Autodesk Fusion 360 part; units mm, degrees
note: some values were not read from the file. Set by a fixed rule: which face or edge a step refers to.
(part 5 of 5)
sketch "Sketch1" plane through (0, 0, 0) normal (0, 0, 1) x (1, 0, 0)
  line L0 (-10, 10) -> (10, 10) construction
  line L1 (10, 10) -> (10, -10) construction
  line L2 (10, -10) -> (-10, -10) construction
  line L3 (-10, -10) -> (-10, 10) construction
  circle A0 centre (0, 0) radius 2.5
  line L4 (0, -10) -> (0, -3.9) construction
  line L5 (-10, 0) -> (-3.9, 0) construction
  line L6 (10, 0) -> (3.9, 0) construction
  line L7 (0, 10) -> (0, 3.9) construction
  line L8 (3.9, 3.6) -> (3.9, 0) construction
  line L9 (3.9, -3.0515) -> (3.9, 3.1)
  line L10 (-3.9, 3.1) -> (-3.9, -3.0515)
  line L11 (10, 10) -> (-10, -10) construction
  line L12 (-10, 10) -> (10, -10) construction
  line L13 (3.9, 3.9) -> (4.3243, 3.4757) construction
  line L14 (3.9, 3.9) -> (3.4757, 4.3243) construction
  line L15 (-3.9, 3.9) -> (-3.4757, 4.3243) construction
  line L16 (-3.4757, 4.3243) -> (-4.3243, 3.4757) construction
  line L17 (-3.9, -3.9) -> (-4.3243, -3.4757) construction
  line L18 (-4.3243, -3.4757) -> (-3.4757, -4.3243) construction
  line L19 (3.9, -3.9) -> (4.3243, -3.4757) construction
  line L20 (4.3243, -3.4757) -> (3.4757, -4.3243) construction
  line L21 (3.4757, -4.3243) -> (3.0515, -3.9)
  line L22 (4.3243, -3.4757) -> (3.9, -3.0515)
  line L23 (10, -10) -> (9.1515, -10)
  line L24 (10, -9.1515) -> (10, -10)
  line L25 (3.4757, 4.3243) -> (3.0515, 3.9)
  line L26 (3.4757, 4.3243) -> (2.8757, 4.3243) construction
  line L27 (4.3243, 3.4757) -> (3.9, 3.0515)
  line L28 (-4.3243, 3.4757) -> (-3.9, 3.0515)
  line L29 (-3.4757, 4.3243) -> (-3.0515, 3.9)
  line L30 (-3.4757, -4.3243) -> (-3.0515, -3.9)
  line L31 (-4.3243, -3.4757) -> (-3.9, -3.0515)
  line L32 (-4.3243, -3.4757) -> (-3.7243, -3.4757) construction
  line L33 (-9.1515, -10) -> (-10, -10)
  line L34 (-10, -10) -> (-10, -9.1515)
  line L35 (-10, 9.1515) -> (-10, 10)
  line L36 (-10, 10) -> (-9.1515, 10)
  line L37 (9.1515, 10) -> (10, 10)
  line L38 (10, 9.1515) -> (10, 10)
  line L39 (10, -10) -> (8.2, -10) construction
  line L40 (8.2, -10) -> (8.2, -8.2) construction
  line L41 (8.2, -8.2) -> (10, -8.2) construction
  line L42 (10, -8.2) -> (10, -10) construction
  line L43 (-10, -10) -> (-8.2, -10) construction
  line L44 (-8.2, -10) -> (-8.2, -8.2) construction
  line L45 (-8.2, -8.2) -> (-10, -8.2) construction
  line L46 (-10, -8.2) -> (-10, -10) construction
  line L47 (-10, 10) -> (-8.2, 10) construction
  line L48 (-8.2, 10) -> (-8.2, 8.2) construction
  line L49 (-8.2, 8.2) -> (-10, 8.2) construction
  line L50 (-10, 8.2) -> (-10, 10) construction
  line L51 (10, 10) -> (8.2, 10) construction
  line L52 (8.2, 10) -> (8.2, 8.2) construction
  line L53 (8.2, 8.2) -> (10, 8.2) construction
  line L54 (10, 8.2) -> (10, 10) construction
  line L55 (-10, -10) -> (-9.1, -10) construction
  line L56 (-9.1, -10) -> (-9.1, -9.1) construction
  line L57 (-9.1, -9.1) -> (-10, -9.1) construction
  line L58 (-10, -9.1) -> (-10, -10) construction
  line L59 (-10, 10) -> (-9.1, 10) construction
  line L60 (-9.1, 10) -> (-9.1, 9.1) construction
  line L61 (-9.1, 9.1) -> (-10, 9.1) construction
  line L62 (-10, 9.1) -> (-10, 10) construction
  line L63 (10, 10) -> (9.1, 10) construction
  line L64 (9.1, 10) -> (9.1, 9.1) construction
  line L65 (9.1, 9.1) -> (10, 9.1) construction
  line L66 (10, 9.1) -> (10, 10) construction
  line L67 (10, -10) -> (9.1, -10) construction
  line L68 (9.1, -10) -> (9.1, -9.1) construction
  line L69 (9.1, -9.1) -> (10, -9.1) construction
  line L70 (10, -9.1) -> (10, -10) construction
  line L71 (0, -10) -> (3.1, -10) construction
  line L72 (3.1, -10) -> (-3, -10) construction
  line L73 (-3, -10) -> (-3, 10) construction
  line L74 (-3, 10) -> (3.1, 10) construction
  line L75 (3.1, 10) -> (3.1, -10) construction
  line L76 (-10, 0) -> (-10, 3.1) construction
  line L77 (-10, 3.1) -> (10, 3.1) construction
  line L78 (10, 3.1) -> (10, -3) construction
  line L79 (10, -3) -> (-10, -3) construction
  line L80 (-10, -3) -> (-10, 3.1) construction
  line L81 (0, -10) -> (-5.45, -10) construction
  line L82 (-5.45, -10) -> (5.45, -10) construction
  line L83 (5.45, 10) -> (-5.45, 10) construction
  line L84 (-10, 0) -> (-10, 5.45) construction
  line L85 (10, 5.45) -> (10, -5.45) construction
  line L86 (-10, -5.45) -> (-10, 5.45) construction
  line L87 (-10, -10) -> (-5.45, -10)
  line L88 (-10, -5.45) -> (-10, -10)
  line L89 (10, -10) -> (5.45, -10)
  line L90 (10, -5.45) -> (10, -10)
  line L91 (10, 10) -> (5.45, 10)
  line L92 (5.45, 8.2) -> (5.45, 6.2985)
  line L93 (10, 5.45) -> (10, 10)
  line L94 (-10, 10) -> (-5.45, 10)
  line L95 (-5.45, 8.2) -> (-5.45, 6.2985)
  line L96 (-6.2985, 5.45) -> (-8.2, 5.45)
  line L97 (-10, 5.45) -> (-10, 10)
  line L98 (10, 0) -> (10, 3.6) construction
  line L99 (-10, 3.6) -> (-10, -3.6) construction
  line L100 (10, -3.6) -> (10, 3.6) construction
  line L101 (0, 10) -> (-3.6, 10) construction
  line L102 (-3.6, 10) -> (3.6, 10) construction
  line L103 (3.6, -10) -> (-3.6, -10) construction
  line L104 (-8.2, -8.2) -> (8.2, -8.2) construction
  line L105 (8.2, -8.2) -> (8.2, 8.2) construction
  line L106 (8.2, 8.2) -> (-8.2, 8.2) construction
  line L107 (-8.2, 8.2) -> (-8.2, -8.2) construction
  line L108 (-5.45, -10) -> (-3.6, -10)
  line L109 (-3.6, -10) -> (-3.6, -9.1)
  line L110 (-3.6, -8.2) -> (-5.45, -8.2)
  line L111 (-10, -3.6) -> (-9.1, -3.6)
  line L112 (-8.2, -3.6) -> (-8.2, -5.45)
  line L113 (-10, -5.45) -> (-10, -3.6)
  line L114 (-9.1, 3.6) -> (-10, 3.6)
  line L115 (-10, 3.6) -> (-10, 5.45)
  line L116 (-8.2, 5.45) -> (-8.2, 3.6)
  line L117 (3.6, 8.2) -> (5.45, 8.2)
  line L118 (5.45, 10) -> (3.6, 10)
  line L119 (3.6, 10) -> (3.6, 9.1)
  line L120 (-5.45, 10) -> (-3.6, 10)
  line L121 (-3.6, 10) -> (-3.6, 9.1)
  line L122 (-3.6, 8.2) -> (-5.45, 8.2)
  line L123 (10, 5.45) -> (10, 3.6)
  line L124 (10, 3.6) -> (9.1, 3.6)
  line L125 (8.2, 3.6) -> (8.2, 5.45)
  line L126 (10, -5.45) -> (10, -3.6)
  line L127 (10, -3.6) -> (9.1, -3.6)
  line L128 (8.2, -3.6) -> (8.2, -5.45)
  line L129 (5.45, -8.2) -> (3.6, -8.2)
  line L130 (3.6, -9.1) -> (3.6, -10)
  line L131 (3.6, -10) -> (5.45, -10)
  line L132 (9.1, -9.1) -> (-9.1, -9.1) construction
  line L133 (-9.1, -9.1) -> (-9.1, 9.1) construction
  line L134 (-9.1, 9.1) -> (9.1, 9.1) construction
  line L135 (9.1, 9.1) -> (9.1, -9.1) construction
  line L136 (3.6, -9.1) -> (3.1, -9.1)
  line L137 (3.1, -9.1) -> (3.1, -8.2)
  line L138 (3.1, -8.2) -> (3.6, -8.2)
  line L139 (-3, -9.1) -> (-3.6, -9.1)
  line L140 (-3.6, -8.2) -> (-3, -8.2)
  line L141 (-3, -8.2) -> (-3, -9.1)
  line L142 (-8.2, -3.6) -> (-8.2, -3)
  line L143 (-8.2, -3) -> (-9.1, -3)
  line L144 (-9.1, -3) -> (-9.1, -3.6)
  line L145 (-8.2, 3.6) -> (-8.2, 3.1)
  line L146 (-8.2, 3.1) -> (-9.1, 3.1)
  line L147 (-9.1, 3.1) -> (-9.1, 3.6)
  line L148 (-3.6, 9.1) -> (-3, 9.1)
  line L149 (-3, 9.1) -> (-3, 8.2)
  line L150 (-3, 8.2) -> (-3.6, 8.2)
  line L151 (3.1, 9.1) -> (3.6, 9.1)
  line L152 (3.6, 8.2) -> (3.1, 8.2)
  line L153 (3.1, 8.2) -> (3.1, 9.1)
  line L154 (9.1, 3.6) -> (9.1, 3.1)
  line L155 (9.1, 3.1) -> (8.2, 3.1)
  line L156 (8.2, 3.1) -> (8.2, 3.6)
  line L157 (9.1, -3.6) -> (9.1, -3)
  line L158 (9.1, -3) -> (8.2, -3)
  line L159 (8.2, -3) -> (8.2, -3.6)
  line L160 (-3.4757, 4.3243) -> (-5.45, 6.2985)
  line L161 (-4.3243, 3.4757) -> (-6.2985, 5.45)
  line L162 (-3.6, 9.1) -> (-3.6, 10) construction
  line L163 (-9.1, 3.6) -> (-10, 3.6) construction
  line L164 (-3.0515, -3.9) -> (3.1, -3.9)
  line L165 (-3.9, 0) -> (-3.9, -3.0515) construction
  line L166 (0, 3.9) -> (3.1, 3.9) construction
  line L167 (3.1, 3.9) -> (-3.0515, 3.9)
  line L168 (-4.3243, -3.4757) -> (-6.2985, -5.45)
  line L169 (-3.4757, -4.3243) -> (-5.45, -6.2985)
  line L170 (-6.2985, -5.45) -> (-8.2, -5.45)
  line L171 (-10, -3.6) -> (-9.1, -3.6) construction
  line L172 (-5.45, -8.2) -> (-5.45, -6.2985)
  line L173 (-3.6, -10) -> (-3.6, -9.1) construction
  line L174 (-3.6, -8.2) -> (-3.6, 8.2) construction
  line L175 (6.2985, -5.45) -> (8.2, -5.45)
  line L176 (-8.2, -3.6) -> (8.2, -3.6) construction
  line L177 (9.1, -3.6) -> (10, -3.6) construction
  line L178 (3.4757, -4.3243) -> (5.45, -6.2985)
  line L179 (8.2, -9.0485) -> (8.2515, -9.1)
  line L180 (9.1, -9.9485) -> (9.1515, -10)
  line L181 (9.9485, -9.1) -> (10, -9.1515)
  line L182 (4.3243, -3.4757) -> (6.2985, -5.45)
  line L183 (9.0485, -8.2) -> (9.1, -8.2515)
  line L184 (5.45, -8.2) -> (5.45, -6.2985)
  line L185 (6.2985, 5.45) -> (8.2, 5.45)
  line L186 (10, 3.6) -> (9.1, 3.6) construction
  line L187 (8.2, 3.6) -> (-8.2, 3.6) construction
  line L188 (3.4757, 4.3243) -> (5.45, 6.2985)
  line L189 (4.3243, 3.4757) -> (6.2985, 5.45)
  line L190 (3.6, 10) -> (3.6, 9.1) construction
  line L191 (3.6, 8.2) -> (3.6, -10) construction
  dimension "d1" = 20
  dimension "d2" = 20
  dimension "d3" = 5
  dimension "d4" = 6.1
  dimension "d5" = 6.1
  dimension "d6" = 6.1
  dimension "d7" = 6.1
  dimension "d8" = 0.6
  dimension "d9" = 0.6
  dimension "d10" = 0.6
  dimension "d11" = 1.2
  dimension "d12" = 0.6
  dimension "d13" = 1.2
  dimension "d14" = 0.6
  dimension "d15" = 1.2
  dimension "d18" = 45
  dimension "d20" = 45
  dimension "d24" = 1.8
  dimension "d25" = 1.8
  dimension "d26" = 1.8
  dimension "d27" = 1.8
  dimension "d28" = 1.8
  dimension "d29" = 1.8
  dimension "d30" = 1.8
  dimension "d31" = 1.8
  dimension "d32" = 0.9
  dimension "d33" = 0.9
  dimension "d34" = 0.9
  dimension "d35" = 0.9
  dimension "d36" = 0.9
  dimension "d37" = 0.9
  dimension "d38" = 0.9
  dimension "d39" = 0.9
  dimension "d40" = 3.1
  dimension "d41" = 6.1
  dimension "d42" = 3.1
  dimension "d43" = 20
  dimension "d44" = 6.1
  dimension "d47" = 5.45
  dimension "d48" = 10.9
  dimension "d49" = 3.6
  dimension "d50" = 7.2
  dimension "d51" = 20
  dimension "d52" = 3.6
  dimension "d53" = 7.2
  dimension "d54" = 20
  constraint horizontal L0
  constraint vertical L1
  constraint horizontal L2
  constraint vertical L3
  constraint coincident A0.centre origin
  constraint midpoint L2 L4.start
  constraint perpendicular L2 L4
  constraint midpoint L3 L5.start
  constraint perpendicular L3 L5
  constraint perpendicular L5 L165
  constraint midpoint L1 L6.start
  constraint perpendicular L1 L6
  constraint midpoint L0 L7.start
  constraint perpendicular L0 L7
  constraint perpendicular L7 L166
  constraint perpendicular L6 L8
  constraint vertical L9
  constraint vertical L10
  constraint parallel L12 L13
  constraint perpendicular L11 L14
  constraint perpendicular L12 L15
  constraint perpendicular L12 L16
  constraint perpendicular L11 L17
  constraint perpendicular L11 L18
  constraint perpendicular L12 L19
  constraint perpendicular L12 L20
  constraint coincident L2 L23.end
  constraint perpendicular L20 L178
  constraint perpendicular L20 L21
  constraint perpendicular L19 L22
  constraint coincident L1 L24.start
  constraint perpendicular L19 L182
  constraint perpendicular L1 L23
  constraint perpendicular L2 L24
  constraint coincident L1 L38.start
  constraint coincident L0 L37.start
  constraint horizontal L26
  constraint coincident L25.end L166
  constraint coincident L8 L27.end
  constraint coincident L10 L28.end
  constraint perpendicular L16 L28
  constraint perpendicular L16 L29
  constraint perpendicular L18 L30
  constraint horizontal L32
  constraint coincident L3 L34.end
  constraint perpendicular L17 L168
  constraint coincident L2 L33.start
  constraint perpendicular L33 L34
  constraint coincident L3 L35.start
  constraint coincident L0 L36.end
  constraint horizontal L39
  constraint vertical L40
  constraint horizontal L41
  constraint vertical L42
  constraint horizontal L43
  constraint vertical L44
  constraint horizontal L45
  constraint vertical L46
  constraint horizontal L47
  constraint vertical L48
  constraint horizontal L49
  constraint vertical L50
  constraint horizontal L51
  constraint vertical L52
  constraint horizontal L53
  constraint vertical L54
  constraint horizontal L55
  constraint vertical L56
  constraint horizontal L57
  constraint vertical L58
  constraint horizontal L59
  constraint vertical L60
  constraint horizontal L61
  constraint vertical L62
  constraint horizontal L63
  constraint vertical L64
  constraint horizontal L65
  constraint vertical L66
  constraint horizontal L67
  constraint vertical L68
  constraint horizontal L69
  constraint vertical L70
  constraint coincident L2 L71.end
  constraint horizontal L72
  constraint vertical L73
  constraint horizontal L74
  constraint vertical L75
  constraint coincident L0 L73.end
  constraint perpendicular L5 L76
  constraint horizontal L77
  constraint vertical L78
  constraint horizontal L79
  constraint vertical L80
  constraint coincident L2 L81.end
  constraint horizontal L82
  constraint horizontal L83
  constraint coincident L0 L83.start
  constraint perpendicular L5 L84
  constraint vertical L85
  constraint vertical L86
  constraint coincident L1 L85.end
  constraint horizontal L87
  constraint horizontal L170
  constraint vertical L88
  constraint horizontal L89
  constraint horizontal L175
  constraint vertical L90
  constraint horizontal L91
  constraint vertical L92
  constraint horizontal L185
  constraint vertical L93
  constraint horizontal L94
  constraint vertical L95
  constraint horizontal L96
  constraint vertical L97
  constraint coincident L85 L98.end
  constraint horizontal L186
  constraint vertical L99
  constraint horizontal L171
  constraint vertical L100
  constraint perpendicular L7 L101
  constraint horizontal L102
  constraint vertical L190
  constraint horizontal L103
  constraint vertical L173
  constraint horizontal L108
  constraint vertical L109
  constraint horizontal L110
  constraint coincident L110.start L173
  constraint coincident L104 L110.start
  constraint horizontal L111
  constraint vertical L112
  constraint vertical L113
  constraint coincident L107 L112.end
  constraint horizontal L114
  constraint vertical L115
  constraint vertical L116
  constraint coincident L107 L116.end
  constraint horizontal L117
  constraint horizontal L118
  constraint vertical L119
  constraint coincident L117.start L190
  constraint coincident L106 L117.start
  constraint horizontal L120
  constraint vertical L121
  constraint horizontal L122
  constraint coincident L106 L122.start
  constraint vertical L123
  constraint horizontal L124
  constraint vertical L125
  constraint coincident L105 L125.end
  constraint vertical L126
  constraint horizontal L127
  constraint vertical L128
  constraint coincident L105 L128.end
  constraint horizontal L129
  constraint vertical L130
  constraint horizontal L131
  constraint coincident L104 L129.start
  constraint horizontal L136
  constraint vertical L137
  constraint horizontal L138
  constraint coincident L75 L137.end
  constraint coincident L104 L137.end
  constraint horizontal L139
  constraint horizontal L140
  constraint vertical L141
  constraint coincident L73 L139.start
  constraint coincident L132 L139.start
  constraint vertical L142
  constraint horizontal L143
  constraint vertical L144
  constraint coincident L107 L142.end
  constraint coincident L79 L142.end
  constraint vertical L145
  constraint horizontal L146
  constraint vertical L147
  constraint coincident L107 L145.end
  constraint coincident L77 L145.end
  constraint horizontal L148
  constraint vertical L149
  constraint horizontal L150
  constraint coincident L73 L149.end
  constraint coincident L106 L149.end
  constraint horizontal L151
  constraint horizontal L152
  constraint vertical L153
  constraint coincident L75 L151.start
  constraint coincident L134 L151.start
  constraint vertical L154
  constraint horizontal L155
  constraint vertical L156
  constraint coincident L135 L154.end
  constraint coincident L77 L154.end
  constraint vertical L157
  constraint horizontal L158
  constraint vertical L159
  constraint coincident L135 L157.end
  constraint coincident L79 L157.end
  constraint coincident L77 L10.start
  constraint collinear L162 L173
  constraint collinear L163 L186
  constraint coincident L75 L164.end
  constraint coincident L75 L166.end
  constraint coincident L8.start L186
  constraint coincident L77 L9.end
  constraint collinear L171 L176
  constraint collinear L173 L174
  constraint collinear L176 L177
  constraint coincident L40 L179.start
  constraint collinear L178 L179
  constraint coincident L132 L179.end
  constraint coincident L68 L180.start
  constraint collinear L179 L180
  constraint coincident L135 L183.end
  constraint coincident L69 L181.start
  constraint collinear L181 L182
  constraint coincident L41 L183.start
  constraint collinear L182 L183
  constraint collinear L186 L187
  constraint collinear L190 L191
  measures "d1" distance of L0.start L0.end
  measures "d2" distance of L0.start L2.end
  measures "d3" diameter of A0
  measures "d4" distance of L4.start L4.end
  measures "d5" distance of L5.start L5.end
  measures "d6" distance of L6.start L6.end
  measures "d7" distance of L7.start L7.end
  measures "d8" distance of L13.start L13.end
  measures "d9" distance of L13.start L14.end
  measures "d10" distance of L15.start L15.end
  measures "d11" distance of L15.end L16.end
  measures "d12" distance of L17.start L17.end
  measures "d13" distance of L17.end L18.end
  measures "d14" distance of L19.start L19.end
  measures "d15" distance of L19.end L20.end
  measures "d18" angle of L25 L26
  measures "d20" angle of L31 L32
  measures "d24" distance of L1.end L39.end
  measures "d25" distance of L1.end L41.end
  measures "d26" distance of L2.end L45.end
  measures "d27" distance of L2.end L43.end
  measures "d28" distance of L0.start L47.end
  measures "d29" distance of L0.start L49.end
  measures "d30" distance of L0.end L53.end
  measures "d31" distance of L0.end L51.end
  measures "d32" distance of L2.end L57.end
  measures "d33" distance of L2.end L55.end
  measures "d34" distance of L0.start L59.end
  measures "d35" distance of L0.start L61.end
  measures "d36" distance of L0.end L63.end
  measures "d37" distance of L0.end L65.end
  measures "d38" distance of L1.end L67.end
  measures "d39" distance of L1.end L69.end
  measures "d40" distance of L4.start L71.end
  measures "d41" distance of L71.end L72.end
  measures "d42" distance of L5.start L76.end
  measures "d43" distance of L76.end L77.end
  measures "d44" distance of L76.end L79.end
  measures "d47" distance of L5.start L84.end
  measures "d48" distance of L84.end L86.start
  measures "d49" distance of L6.start L98.end
  measures "d50" distance of L98.end L100.start
  measures "d51" distance of L98.end L99.start
  measures "d52" distance of L7.start L101.end
  measures "d53" distance of L101.end L102.end
  measures "d54" distance of L101.end L103.end
extrude "Extrude1" add sketch "Sketch1" along normal blind 433.8491 makes body 1
delete_body "RemoveBody1" bodies 1
sketch "Sketch2" plane through (0, 0, 0) normal (0, 1, 0) x (1, 0, 0)
  line L0 (-10, -10) -> (10, -10)
  line L1 (10, -10) -> (10, 10)
  line L2 (10, 10) -> (-10, 10)
  line L3 (-10, 10) -> (-10, -10)
  line L4 (-10, -10) -> (10, 10) construction
  line L5 (10, -10) -> (-10, 10) construction
  line L6 (0, 0) -> (15.5296, -8.0673) construction
  line L7 (0, 0) -> (17.5, 0) construction
  line L8 (15.5296, -8.0673) -> (51.0258, -26.5069) construction
  line L9 (44.111, -39.818) -> (57.9407, -13.1958)
  line L10 (15, 15) -> (-15, 15)
  line L11 (-15, 15) -> (-15, -15)
  line L12 (-15, -15) -> (15, -15)
  line L13 (15, -15) -> (15, 15)
  line L14 (15, 15) -> (-15, -15) construction
  line L15 (-15, 15) -> (15, -15) construction
  line L16 (10.15, -10.15) -> (10.15, 10.15)
  line L17 (10.15, 10.15) -> (-10.15, 10.15)
  line L18 (-10.15, 10.15) -> (-10.15, -10.15)
  line L19 (-10.15, -10.15) -> (10.15, -10.15)
  line L20 (57.9407, -13.1958) -> (15, 9.111)
  line L21 (44.111, -39.818) -> (-3.6637, -15)
  circle A0 centre (33.2777, -17.2871) radius 1.5
  circle A1 centre (33.2777, -17.2871) radius 1.8
  dimension "d63" = 20
  dimension "d64" = 20
  dimension "d65" = 27.451
  dimension "d66" = 17.5
  dimension "d67" = 40
  dimension "d68" = 30
  dimension "d69" = 30
  dimension "d70" = 30
  dimension "d71" = 0.15
  dimension "d72" = 3
  dimension "d73" = 0.3
  constraint horizontal L0
  constraint perpendicular L0 L1
  constraint parallel L0 L2
  constraint parallel L1 L3
  constraint coincident L4 L6.start
  constraint coincident L5 L6.start
  constraint coincident L6.start L7.start
  constraint horizontal L7
  constraint parallel L6 L8
  constraint midpoint L8.end L9
  constraint perpendicular L8 L9
  constraint horizontal L10
  constraint perpendicular L10 L11
  constraint parallel L10 L12
  constraint parallel L11 L13
  constraint coincident L14 L6.start
  constraint coincident L15 L6.start
  constraint coincident L13 L20.end
  constraint perpendicular L9 L20
  constraint coincident L12 L21.end
  constraint perpendicular L9 L21
  constraint midpoint L8 A0.centre
  measures "d63" distance of L1.end L2.end
  measures "d64" distance of L0.end L1.end
  measures "d65" angle of L6 L7
  measures "d66" distance of L6.start L6.end
  measures "d67" distance of L6.end L8.end
  measures "d68" distance of L9.start L9.end
  measures "d69" distance of L11.end L12.end
  measures "d70" distance of L10.end L11.end
  measures "d72" diameter of A0
extrude "Extrude2" add sketch "Sketch2" along normal mid plane 60 separate body contours L10 L11 L12 L13 makes body 2
extrude "Extrude3" add sketch "Sketch2" along normal mid plane 30 contours L9 L12 L13 L20 L21 bodies 2
sketch "Sketch3" plane through (51.0258, 0, 26.5069) normal (0.887405, 0, 0.46099) x (0, 1, 0)
  line L0 (-15, -15) -> (15, -15)
  line L1 (15, -15) -> (15, 15)
  line L2 (15, 15) -> (-15, 15)
  line L3 (-15, 15) -> (-15, -15)
  line L4 (-10, 10) -> (10, 10)
  line L5 (10, 10) -> (10, -10)
  line L6 (10, -10) -> (-10, -10)
  line L7 (-10, -10) -> (-10, 10)
  line L8 (-10, 10) -> (10, -10) construction
  line L9 (10, 10) -> (-10, -10) construction
  line L10 (10.15, -10.15) -> (-10.15, -10.15)
  line L11 (-10.15, -10.15) -> (-10.15, 10.15)
  line L12 (-10.15, 10.15) -> (10.15, 10.15)
  line L13 (10.15, 10.15) -> (10.15, -10.15)
  dimension "d78" = 20
  dimension "d79" = 20
  dimension "d80" = -0.15
  constraint horizontal L4
  constraint perpendicular L4 L5
  constraint parallel L4 L6
  constraint parallel L5 L7
  constraint coincident L8 origin
  constraint coincident L9 origin
  measures "d78" distance of L5.end L6.end
  measures "d79" distance of L4.end L5.end
extrude "Extrude4" cut sketch "Sketch3" against normal blind 40 contours L4 L5 L6 L7 | L10 L11 L12 L13 bodies 2
sketch "Sketch4" plane through (-15, 0, 0) normal (-1, 0, 0) x (0, -1, 0)
  line L0 (30, 15) -> (-30, 15)
  line L1 (-30, 15) -> (-30, -15)
  line L2 (-30, -15) -> (30, -15)
  line L3 (30, -15) -> (30, 15)
  line L4 (0, 0) -> (30, 0) construction
  line L5 (0, 0) -> (-30, 0) construction
  circle A0 centre (15, 0) radius 1.65
  circle A1 centre (-15, 0) radius 1.65
  dimension "d83" = 3.3
  dimension "d84" = 3.3
  constraint coincident L4.start L5.start
  constraint midpoint L3 L4.end
  constraint midpoint L1 L5.end
  constraint midpoint L4 A0.centre
  constraint midpoint L5 A1.centre
  measures "d83" diameter of A0
  measures "d84" diameter of A1
extrude "Extrude5" cut sketch "Sketch4" against normal blind 13 contours A0 | A1 bodies 2
equation "socketlength = 40 mm"
equation "angle = atan(h / ( 520 mm - distFromEdge ))"
equation "distFromEdge = 135 mm"
equation "length = 1 / sin(angle) * h"
equation "d61 = length"
equation "d65 = angle"
equation "d67 = socketlength"
